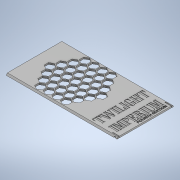
# Autodesk Inventor part: CardboardTray_Lid2
Saved by Autodesk Inventor 2021 (Build 250183000, 183)
## iProperties
Created: 2023-03-19
Part Number: CardboardTray_Lid2
Material: ABS Plastic
Document SubType Name: Modeling
Designer: Bradley
Density: 1.06 g/cm^3
Appearance: Smooth - Medium Gray
Author: Bradley
Autodesk Inventor part; units mm, degrees
(part 1 of 2)
ref_plane "YZ Plane" through (0, 0, 0) normal (1, 0, 0) x (0, 1, 0)
ref_plane "XZ Plane" through (0, 0, 0) normal (0, 1, 0) x (-1, 0, 0)
ref_plane "XY Plane" through (0, 0, 0) normal (0, 0, 1) x (1, 0, 0)
sketch "Sketch1" plane through (0, 0, 0) normal (1, 0, 0) x (0, 1, 0)
  line L0 (-1, 36.1) -> (-1, -36.1)
  line L1 (-1, -36.1) -> (1, -34.6)
  line L2 (1, -34.6) -> (1, 34.6)
  line L3 (1, 34.6) -> (-1, 36.1)
  point P0 (0, 0)
  point P1 (0, 35.35)
  point P2 (1, 0)
  dimension "d0" = 2
  dimension "d1" = 1.5
  dimension "d2" = 69.2
  constraints: 8 end point, 2 midpoint, 1 equal length, 1 horizontal alignment, 1 parallel, 1 vertical, 1 vertical alignment
  measures "d0" distance between parallel lines of L0 L2
  measures "d1" vertical distance of L2.end L0.start
  measures "d2" distance of L1.end L2.end
extrude "Extrusion1" add sketch "Sketch1" along normal mid plane 140.85
sketch "Sketch2" plane through (-70.425, 1, 34.6) normal (0, 1, 0) x (1, 0, 0)
  line L0 (0, 0) -> (140.85, 0) projected
  line L1 (140.85, 69.2) -> (140.85, 0) projected
  line L2 (0, 69.2) -> (140.85, 69.2) projected
  line L3 (0, 0) -> (0, 69.2) projected
  line L4 (0, 69.2) -> (140.85, 69.2) projected
  line L5 (140.85, 70.7) -> (140.85, 69.2) projected
  line L6 (140.85, 70.7) -> (0, 70.7) projected
  line L7 (0, 69.2) -> (0, 70.7) projected
  line L8 (0, -1.5) -> (140.85, -1.5) projected
  line L9 (140.85, 0) -> (140.85, -1.5) projected
  line L10 (0, 0) -> (140.85, 0) projected
  line L11 (0, -1.5) -> (0, 0) projected
  line L12 (140.85, 70.7) -> (0, 70.7) projected
  line L13 (139.1, 70.7) -> (138.8979, 70.35) construction
  line L14 (138.4649, 70.1) -> (137.2351, 70.1) construction
  line L15 (136.8021, 70.35) -> (136.6, 70.7) construction
  arc A0 (138.4649, 70.1) -> (138.8979, 70.35) centre (138.4649, 70.6) ccw construction
  arc A1 (136.8021, 70.35) -> (137.2351, 70.1) centre (137.2351, 70.6) ccw construction
  line L16 (140.35, 70.7) -> (140.85, 70.2)
  line L17 (140.85, 70.7) -> (140.85, 69.2) projected
  line L18 (136.3113, 70.7) -> (136.5856, 70.225)
  arc A2 (136.5856, 70.225) -> (137.2351, 69.85) centre (137.2351, 70.6) ccw
  line L19 (137.2351, 69.85) -> (138.2762, 69.85)
  line L20 (138.9258, 70.225) -> (139.2, 70.7)
  line L21 (0, -1.5) -> (140.85, -1.5) projected
  line L22 (140.35, -1.5) -> (140.85, -1)
  line L23 (140.85, 0) -> (140.85, -1.5) projected
  line L24 (139.2, -1.5) -> (138.9258, -1.025)
  arc A3 (138.9258, -1.025) -> (138.2762, -0.65) centre (138.2762, -1.4) ccw
  line L25 (138.2762, -0.65) -> (137.2351, -0.65)
  arc A4 (137.2351, -0.65) -> (136.5856, -1.025) centre (137.2351, -1.4) ccw
  line L26 (136.5856, -1.025) -> (136.3113, -1.5)
  arc A5 (138.2762, 69.85) -> (138.9258, 70.225) centre (138.2762, 70.6) ccw
  line L27 (140.85, 69.2) -> (140.85, 0) projected
  line L28 (140.85, 68.35) -> (132.85, 68.35)
  arc A6 (132.85, 68.35) -> (132.85, 67.55) centre (132.85, 67.95) ccw
  line L29 (132.85, 67.55) -> (140.85, 67.55)
  line L30 (140.85, 0.85) -> (132.85, 0.85)
  arc A7 (132.85, 1.65) -> (132.85, 0.85) centre (132.85, 1.25) ccw
  line L31 (132.85, 1.65) -> (140.85, 1.65)
  point P0 (70.425, 34.6)
  point P1 (137.7557, -0.65)
  point P2 (137.7557, 69.85)
  point P3 (137.85, 70.1)
  point P4 (140.85, 1.65)
  point P5 (140.85, -1)
  dimension "d5" = 0.5
  dimension "d6" = 45
  dimension "d7" = 0.5
  dimension "d8" = 0.25
  dimension "d10" = 0.6
  dimension "d11" = 60
  dimension "d12" = 2.5
  dimension "d13" = 3
  dimension "d14" = 0.1
  dimension "d15" = 1.5
  dimension "d16" = 0.8
  dimension "d17" = 8
  dimension "d18" = 1.5
  constraints: 30 end point, 16 point on circle, 14 point on line, 14 tangent, 8 centre point, 5 equal length, 5 equal radius, 5 perpendicular, 3 midpoint, 3 vertical alignment, 2 parallel, 1 horizontal, 2 other
  measures "d5" radius of A0
  measures "d6" angle of L6 L16
  measures "d7" horizontal distance of L16.start L16.end
  measures "d8" distance between parallel lines of L19 L14
  measures "d10" distance between parallel lines of L14 L6
  measures "d11" angle of L13 L15
  measures "d12" distance of L13.start L15.end
  measures "d13" distance from line of L17 point (137.85, 70.1)
  measures "d14" distance of L13.start L20.end
  measures "d15" distance between parallel lines of L28 L19
  measures "d16" distance between parallel lines of L29 L28
  measures "d17" distance of L28.start L28.end
  measures "d18" distance between parallel lines of L25 L30
extrude "Extrusion2" cut sketch "Sketch2" against normal through all contours L30 A7 L31 L1 | L9 L8 L22 | L26 A4 L25 A3 L24 L8 | L1 L29 A6 L28 | L16 L6 L5 | L6 L20 A5 L19 A2 L18
sketch "Sketch4" plane through (-70.425, 1, -34.6) normal (0, 1, 0) x (1, 0, 0)
  line L0 (140.85, -68.35) -> (132.85, -68.35) projected
  arc A0 (132.85, -67.55) -> (132.85, -68.35) centre (132.85, -67.95) ccw projected
  line L1 (132.85, -67.55) -> (140.85, -67.55) projected
  line L2 (140.85, -1.65) -> (140.85, -67.55) projected
  line L3 (140.85, -1.65) -> (132.85, -1.65) projected
  arc A1 (132.85, -0.85) -> (132.85, -1.65) centre (132.85, -1.25) ccw projected
  line L4 (132.85, -0.85) -> (140.85, -0.85) projected
  line L5 (140.85, 0) -> (140.85, -0.85) projected
  line L6 (0, 0) -> (140.85, 0) projected
  line L7 (0, -69.2) -> (0, 0) projected
  line L8 (0, -69.2) -> (140.85, -69.2) projected
  line L9 (140.85, -68.35) -> (140.85, -69.2) projected
  line L10 (140.85, -67.55) -> (140.85, -1.65) construction
  line L11 (115.85, 0) -> (115.85, -69.2) construction
  line L12 (0, 1.5) -> (0, -70.7) construction
  line L13 (0, 0) -> (140.85, 0) projected
  line L14 (138.85, -1.65) -> (138.85, -67.55) construction
  line L15 (108.9603, -58.6209) -> (105.0262, -58.6209)
  spline S0 degree 2 poles (105.0262, -58.6209) (104.9674, -58.6209) (104.9185, -58.6894) (104.9185, -58.7481) knots 0 0 0 1 2 2 2
  line L16 (104.9185, -58.7481) -> (104.9185, -66.499)
  spline S1 degree 2 poles (104.9185, -66.499) (104.9185, -66.5577) (104.9674, -66.6262) (105.0262, -66.6262) knots 0 0 0 1 2 2 2
  line L17 (105.0262, -66.6262) -> (108.9603, -66.6262)
  spline S2 degree 2 poles (108.9603, -66.6262) (109.0386, -66.6262) (109.1071, -66.5577) (109.0973, -66.5186) knots 0 0 0 1 2 2 2
  spline S3 degree 2 poles (109.0973, -66.5186) (109.1071, -66.4697) (109.0484, -66.4109) (108.9603, -66.4109) knots 0 0 0 1 2 2 2
  line L18 (108.9603, -66.4109) -> (108.7157, -66.4109)
  spline S4 degree 2 poles (108.7157, -66.4109) (107.7664, -66.4012) (106.1516, -65.8335) (105.1534, -64.8255) (105.1338, -64.1796) knots 0 0 0 1 2 3 3 3
  line L19 (105.1338, -64.1796) -> (105.1338, -63.8958)
  spline S5 degree 2 poles (105.1338, -63.8958) (105.1338, -63.8273) (105.1827, -63.7784) (105.2121, -63.7784) knots 0 0 0 1 2 2 2
  line L20 (105.2121, -63.7784) -> (115.0671, -63.7784)
  spline S6 degree 2 poles (115.0671, -63.7784) (115.439, -63.7686) (115.6738, -63.8371) (115.6641, -63.9448) knots 0 0 0 1 2 2 2
  line L21 (115.6641, -63.9448) -> (115.6641, -64.4243)
  spline S7 degree 2 poles (115.6641, -64.4243) (115.6641, -64.5026) (115.7228, -64.5711) (115.7619, -64.5613) knots 0 0 0 1 2 2 2
  spline S8 degree 2 poles (115.7619, -64.5613) (115.7913, -64.5711) (115.85, -64.5026) (115.85, -64.4243) knots 0 0 0 1 2 2 2
  line L22 (115.85, -64.4243) -> (115.85, -60.8229)
  spline S9 degree 2 poles (115.85, -60.8229) (115.85, -60.7446) (115.7913, -60.6761) (115.7619, -60.6859) knots 0 0 0 1 2 2 2
  spline S10 degree 2 poles (115.7619, -60.6859) (115.7228, -60.6761) (115.6641, -60.7348) (115.6641, -60.8229) knots 0 0 0 1 2 2 2
  line L23 (115.6641, -60.8229) -> (115.6641, -61.3024)
  spline S11 degree 2 poles (115.6641, -61.3024) (115.6738, -61.4003) (115.439, -61.4688) (115.0671, -61.4688) knots 0 0 0 1 2 2 2
  line L24 (115.0671, -61.4688) -> (105.2121, -61.4688)
  spline S12 degree 2 poles (105.2121, -61.4688) (105.1827, -61.4688) (105.1338, -61.4101) (105.1338, -61.3318) knots 0 0 0 1 2 2 2
  line L25 (105.1338, -61.3318) -> (105.1338, -61.0675)
  spline S13 degree 2 poles (105.1338, -61.0675) (105.1534, -60.4216) (106.1516, -59.4136) (107.7664, -58.846) (108.7157, -58.8362) knots 0 0 0 1 2 3 3 3
  line L26 (108.7157, -58.8362) -> (108.9603, -58.8362)
  spline S14 degree 2 poles (108.9603, -58.8362) (109.0484, -58.8362) (109.1071, -58.7775) (109.0973, -58.7286) knots 0 0 0 1 2 2 2
  spline S15 degree 2 poles (109.0973, -58.7286) (109.1071, -58.6796) (109.0386, -58.6209) (108.9603, -58.6209) knots 0 0 0 1 2 2 2
  spline S16 degree 2 poles (105.0164, -44.7828) (104.9772, -44.7828) (104.9185, -44.8318) (104.9185, -44.9198) knots 0 0 0 1 2 2 2
  line L27 (104.9185, -44.9198) -> (104.9185, -47.3371)
  spline S17 degree 2 poles (104.9185, -47.3371) (104.9185, -47.4154) (104.9772, -47.4643) (105.0164, -47.4643) knots 0 0 0 1 2 2 2
  spline S18 degree 2 poles (105.0164, -47.4643) (105.0457, -47.4643) (105.1044, -47.4154) (105.1044, -47.3371) knots 0 0 0 1 2 2 2
  line L28 (105.1044, -47.3371) -> (105.1044, -47.1512)
  spline S19 degree 2 poles (105.1044, -47.1512) (105.1142, -46.6129) (106.5333, -46.2606) (107.874, -46.5346) knots 0 0 0 1 2 2 2
  line L29 (107.874, -46.5346) -> (113.9319, -47.7873)
  line L30 (113.9319, -47.7873) -> (113.9319, -47.8362)
  line L31 (113.9319, -47.8362) -> (105.7406, -49.6271)
  spline S20 degree 2 poles (105.7406, -49.6271) (105.3295, -49.725) (105.0947, -49.6467) (105.1044, -49.4999) knots 0 0 0 1 2 2 2
  line L32 (105.1044, -49.4999) -> (105.1044, -49.128)
  spline S21 degree 2 poles (105.1044, -49.128) (105.1044, -49.0399) (105.0457, -48.991) (105.0164, -48.991) knots 0 0 0 1 2 2 2
  spline S22 degree 2 poles (105.0164, -48.991) (104.9772, -48.991) (104.9185, -49.0399) (104.9185, -49.128) knots 0 0 0 1 2 2 2
  line L33 (104.9185, -49.128) -> (104.9185, -52.8273)
  spline S23 degree 2 poles (104.9185, -52.8273) (104.9185, -52.9154) (104.9772, -52.9741) (105.0164, -52.9741) knots 0 0 0 1 2 2 2
  spline S24 degree 2 poles (105.0164, -52.9741) (105.0457, -52.9741) (105.1044, -52.9252) (105.1044, -52.8273) knots 0 0 0 1 2 2 2
  line L34 (105.1044, -52.8273) -> (105.1044, -52.6609)
  spline S25 degree 2 poles (105.1044, -52.6609) (105.1142, -52.1129) (106.5333, -51.7802) (107.874, -52.0444) knots 0 0 0 1 2 2 2
  line L35 (107.874, -52.0444) -> (113.9319, -53.2383)
  line L36 (113.9319, -53.2383) -> (113.9319, -53.2775)
  line L37 (113.9319, -53.2775) -> (105.7406, -55.1369)
  spline S26 degree 2 poles (105.7406, -55.1369) (105.3393, -55.225) (105.0947, -55.1565) (105.1044, -55.0097) knots 0 0 0 1 2 2 2
  line L38 (105.1044, -55.0097) -> (105.1044, -54.628)
  spline S27 degree 2 poles (105.1044, -54.628) (105.1044, -54.5399) (105.0457, -54.4812) (105.0164, -54.491) knots 0 0 0 1 2 2 2
  spline S28 degree 2 poles (105.0164, -54.491) (104.9772, -54.4812) (104.9185, -54.5497) (104.9185, -54.628) knots 0 0 0 1 2 2 2
  line L39 (104.9185, -54.628) -> (104.9185, -58.1903)
  spline S29 degree 2 poles (104.9185, -58.1903) (104.9185, -58.2686) (104.9772, -58.3273) (105.0164, -58.3273) knots 0 0 0 1 2 2 2
  spline S30 degree 2 poles (105.0164, -58.3273) (105.0457, -58.3273) (105.1044, -58.2784) (105.1044, -58.1903) knots 0 0 0 1 2 2 2
  line L40 (105.1044, -58.1903) -> (105.1044, -57.9848)
  spline S31 degree 2 poles (105.1044, -57.9848) (105.0947, -57.8576) (105.3393, -57.701) (105.7406, -57.6031) knots 0 0 0 1 2 2 2
  line L41 (105.7406, -57.6031) -> (115.7913, -55.1076)
  spline S32 degree 2 poles (115.7913, -55.1076) (115.8304, -55.1076) (115.8794, -55.0586) (115.8794, -54.9999) knots 0 0 0 1 2 2 2
  line L42 (115.8794, -54.9999) -> (115.8794, -53.5613)
  spline S33 degree 2 poles (115.8794, -53.5613) (115.8794, -53.4928) (115.8304, -53.4439) (115.7913, -53.4341) knots 0 0 0 1 2 2 2
  line L43 (115.7913, -53.4341) -> (107.5413, -51.7019)
  line L44 (107.5413, -51.7019) -> (107.5413, -51.6725)
  line L45 (107.5413, -51.6725) -> (115.7913, -49.6565)
  spline S34 degree 2 poles (115.7913, -49.6565) (115.8304, -49.6565) (115.8794, -49.6076) (115.8794, -49.5488) knots 0 0 0 1 2 2 2
  line L46 (115.8794, -49.5488) -> (115.8794, -48.1102)
  spline S35 degree 2 poles (115.8794, -48.1102) (115.8794, -48.0417) (115.8304, -47.9928) (115.7913, -47.983) knots 0 0 0 1 2 2 2
  line L47 (115.7913, -47.983) -> (108.0306, -46.3193)
  spline S36 degree 2 poles (108.0306, -46.3193) (106.7388, -46.0257) (105.4763, -45.5364) (105.0849, -45.1254) (105.1044, -44.9492) knots 0 0 0 1 2 3 3 3
  line L48 (105.1044, -44.9492) -> (105.1044, -44.9198)
  spline S37 degree 2 poles (105.1044, -44.9198) (105.1044, -44.8318) (105.0457, -44.7828) (105.0164, -44.7828) knots 0 0 0 1 2 2 2
  spline S38 degree 2 poles (115.7619, -40.6921) (115.7228, -40.6823) (115.6641, -40.741) (115.6641, -40.8291) knots 0 0 0 1 2 2 2
  line L49 (115.6641, -40.8291) -> (115.6641, -41.2597)
  spline S39 degree 2 poles (115.6641, -41.2597) (115.6738, -41.3673) (115.439, -41.4163) (115.0671, -41.4163) knots 0 0 0 1 2 2 2
  line L50 (115.0671, -41.4163) -> (105.7112, -41.4163)
  spline S40 degree 2 poles (105.7112, -41.4163) (105.3393, -41.4163) (105.0947, -41.3673) (105.1044, -41.2597) knots 0 0 0 1 2 2 2
  line L51 (105.1044, -41.2597) -> (105.1044, -40.8291)
  spline S41 degree 2 poles (105.1044, -40.8291) (105.1044, -40.741) (105.0457, -40.6823) (105.0164, -40.6921) knots 0 0 0 1 2 2 2
  spline S42 degree 2 poles (105.0164, -40.6921) (104.9772, -40.6921) (104.9185, -40.7508) (104.9185, -40.8291) knots 0 0 0 1 2 2 2
  line L52 (104.9185, -40.8291) -> (104.9185, -44.3229)
  spline S43 degree 2 poles (104.9185, -44.3229) (104.9185, -44.4012) (104.9772, -44.4599) (105.0164, -44.4599) knots 0 0 0 1 2 2 2
  spline S44 degree 2 poles (105.0164, -44.4599) (105.0457, -44.4697) (105.1044, -44.4109) (105.1044, -44.3229) knots 0 0 0 1 2 2 2
  line L53 (105.1044, -44.3229) -> (105.1044, -43.8923)
  spline S45 degree 2 poles (105.1044, -43.8923) (105.0947, -43.7846) (105.3393, -43.7357) (105.7112, -43.7357) knots 0 0 0 1 2 2 2
  line L54 (105.7112, -43.7357) -> (115.0671, -43.7357)
  spline S46 degree 2 poles (115.0671, -43.7357) (115.439, -43.7357) (115.6738, -43.7846) (115.6641, -43.8923) knots 0 0 0 1 2 2 2
  line L55 (115.6641, -43.8923) -> (115.6641, -44.3229)
  spline S47 degree 2 poles (115.6641, -44.3229) (115.6641, -44.4109) (115.7228, -44.4697) (115.7619, -44.4599) knots 0 0 0 1 2 2 2
  spline S48 degree 2 poles (115.7619, -44.4599) (115.7913, -44.4599) (115.85, -44.4012) (115.85, -44.3229) knots 0 0 0 1 2 2 2
  line L56 (115.85, -44.3229) -> (115.85, -40.8291)
  spline S49 degree 2 poles (115.85, -40.8291) (115.85, -40.7508) (115.7913, -40.6921) (115.7619, -40.6921) knots 0 0 0 1 2 2 2
  line L57 (115.7228, -33.2935) -> (111.5929, -33.2935)
  spline S50 degree 2 poles (111.5929, -33.2935) (111.5048, -33.2935) (111.4559, -33.362) (111.4559, -33.4109) knots 0 0 0 1 2 2 2
  spline S51 degree 2 poles (111.4559, -33.4109) (111.4559, -33.4501) (111.5048, -33.5088) (111.5929, -33.5088) knots 0 0 0 1 2 2 2
  line L58 (111.5929, -33.5088) -> (111.8278, -33.5088)
  spline S52 degree 2 poles (111.8278, -33.5088) (112.3367, -33.5088) (113.6187, -33.8122) (114.8322, -34.4777) (115.6249, -35.564) (115.6347, -36.3567) knots 0 0 0 1 2 3 4 4 4
  line L59 (115.6347, -36.3567) -> (115.6347, -36.9439)
  spline S53 degree 2 poles (115.6347, -36.9439) (115.6347, -37.0124) (115.5956, -37.0515) (115.5564, -37.0515) knots 0 0 0 1 2 2 2
  line L60 (115.5564, -37.0515) -> (105.7112, -37.0515)
  spline S54 degree 2 poles (105.7112, -37.0515) (105.3393, -37.0515) (105.0947, -37.0026) (105.1044, -36.8949) knots 0 0 0 1 2 2 2
  line L61 (105.1044, -36.8949) -> (105.1044, -36.1903)
  spline S55 degree 2 poles (105.1044, -36.1903) (105.1044, -36.0924) (105.0457, -36.0435) (105.0164, -36.0435) knots 0 0 0 1 2 2 2
  spline S56 degree 2 poles (105.0164, -36.0435) (104.9772, -36.0435) (104.9185, -36.0924) (104.9185, -36.1903) knots 0 0 0 1 2 2 2
  line L62 (104.9185, -36.1903) -> (104.9185, -39.9581)
  spline S57 degree 2 poles (104.9185, -39.9581) (104.9185, -40.0364) (104.9772, -40.0951) (105.0164, -40.0951) knots 0 0 0 1 2 2 2
  spline S58 degree 2 poles (105.0164, -40.0951) (105.0457, -40.1049) (105.1044, -40.0462) (105.1044, -39.9581) knots 0 0 0 1 2 2 2
  line L63 (105.1044, -39.9581) -> (105.1044, -39.5275)
  spline S59 degree 2 poles (105.1044, -39.5275) (105.0947, -39.4198) (105.3393, -39.3709) (105.7112, -39.3709) knots 0 0 0 1 2 2 2
  line L64 (105.7112, -39.3709) -> (115.0671, -39.3709)
  spline S60 degree 2 poles (115.0671, -39.3709) (115.439, -39.3709) (115.6738, -39.4198) (115.6641, -39.5275) knots 0 0 0 1 2 2 2
  line L65 (115.6641, -39.5275) -> (115.6641, -39.9581)
  spline S61 degree 2 poles (115.6641, -39.9581) (115.6641, -40.0462) (115.7228, -40.1049) (115.7619, -40.0951) knots 0 0 0 1 2 2 2
  spline S62 degree 2 poles (115.7619, -40.0951) (115.7913, -40.0951) (115.85, -40.0364) (115.85, -39.9581) knots 0 0 0 1 2 2 2
  line L66 (115.85, -39.9581) -> (115.85, -33.4109)
  spline S63 degree 2 poles (115.85, -33.4109) (115.85, -33.3522) (115.7913, -33.2935) (115.7228, -33.2935) knots 0 0 0 1 2 2 2
  spline S64 degree 2 poles (115.7619, -28.7917) (115.7228, -28.7819) (115.6641, -28.8407) (115.6641, -28.9287) knots 0 0 0 1 2 2 2
  line L67 (115.6641, -28.9287) -> (115.6641, -29.3593)
  spline S65 degree 2 poles (115.6641, -29.3593) (115.6738, -29.467) (115.439, -29.5159) (115.0671, -29.5159) knots 0 0 0 1 2 2 2
  line L68 (115.0671, -29.5159) -> (105.7112, -29.5159)
  spline S66 degree 2 poles (105.7112, -29.5159) (105.3393, -29.5159) (105.0947, -29.467) (105.1044, -29.3593) knots 0 0 0 1 2 2 2
  line L69 (105.1044, -29.3593) -> (105.1044, -28.9287)
  spline S67 degree 2 poles (105.1044, -28.9287) (105.1044, -28.8407) (105.0457, -28.7819) (105.0164, -28.7917) knots 0 0 0 1 2 2 2
  spline S68 degree 2 poles (105.0164, -28.7917) (104.9772, -28.7917) (104.9185, -28.8504) (104.9185, -28.9287) knots 0 0 0 1 2 2 2
  line L70 (104.9185, -28.9287) -> (104.9185, -32.4225)
  spline S69 degree 2 poles (104.9185, -32.4225) (104.9185, -32.5008) (104.9772, -32.5595) (105.0164, -32.5595) knots 0 0 0 1 2 2 2
  spline S70 degree 2 poles (105.0164, -32.5595) (105.0457, -32.5693) (105.1044, -32.5106) (105.1044, -32.4225) knots 0 0 0 1 2 2 2
  line L71 (105.1044, -32.4225) -> (105.1044, -31.9919)
  spline S71 degree 2 poles (105.1044, -31.9919) (105.0947, -31.8843) (105.3393, -31.8353) (105.7112, -31.8353) knots 0 0 0 1 2 2 2
  line L72 (105.7112, -31.8353) -> (115.0671, -31.8353)
  spline S72 degree 2 poles (115.0671, -31.8353) (115.439, -31.8353) (115.6738, -31.8843) (115.6641, -31.9919) knots 0 0 0 1 2 2 2
  line L73 (115.6641, -31.9919) -> (115.6641, -32.4225)
  spline S73 degree 2 poles (115.6641, -32.4225) (115.6641, -32.5106) (115.7228, -32.5693) (115.7619, -32.5595) knots 0 0 0 1 2 2 2
  spline S74 degree 2 poles (115.7619, -32.5595) (115.7913, -32.5595) (115.85, -32.5008) (115.85, -32.4225) knots 0 0 0 1 2 2 2
  line L74 (115.85, -32.4225) -> (115.85, -28.9287)
  spline S75 degree 2 poles (115.85, -28.9287) (115.85, -28.8504) (115.7913, -28.7917) (115.7619, -28.7917) knots 0 0 0 1 2 2 2
  spline S76 degree 2 poles (111.2406, -20.1013) (111.2014, -20.0915) (111.1427, -20.1601) (111.1427, -20.2383) knots 0 0 0 1 2 2 2
  line L75 (111.1427, -20.2383) -> (111.1427, -24.0746)
  spline S77 degree 2 poles (111.1427, -24.0746) (111.1427, -24.1725) (111.2014, -24.2214) (111.2406, -24.2214) knots 0 0 0 1 2 2 2
  spline S78 degree 2 poles (111.2406, -24.2214) (111.2699, -24.2214) (111.3286, -24.1725) (111.3286, -24.0746) knots 0 0 0 1 2 2 2
  line L76 (111.3286, -24.0746) -> (111.3286, -23.2428)
  spline S79 degree 2 poles (111.3286, -23.2428) (111.3189, -23.1351) (111.5635, -23.0764) (111.9354, -23.0862) knots 0 0 0 1 2 2 2
  line L77 (111.9354, -23.0862) -> (114.1961, -23.0862)
  spline S80 degree 2 poles (114.1961, -23.0862) (114.9888, -23.0666) (115.8598, -23.4972) (115.8696, -24.1431) knots 0 0 0 1 2 2 2
  spline S81 degree 2 poles (115.8696, -24.1431) (115.8598, -24.7108) (115.0769, -25.2099) (113.648, -25.3371) (112.6792, -25.3665) knots 0 0 0 1 2 3 3 3
  spline S82 degree 2 poles (112.6792, -25.3665) (111.544, -25.4154) (109.2833, -25.4154) (108.1578, -25.3665) knots 0 0 0 1 2 2 2
  spline S83 degree 2 poles (108.1578, -25.3665) (107.2966, -25.3469) (105.8286, -25.2001) (104.9185, -24.6716) (104.9087, -24.0942) knots 0 0 0 1 2 3 3 3
  spline S84 degree 2 poles (104.9087, -24.0942) (104.9185, -23.5462) (105.8286, -22.4403) (107.5315, -21.6867) (108.7352, -21.677) knots 0 0 0 1 2 3 3 3
  line L78 (108.7352, -21.677) -> (108.9016, -21.677)
  spline S85 degree 2 poles (108.9016, -21.677) (108.9897, -21.677) (109.0386, -21.6182) (109.0386, -21.5791) knots 0 0 0 1 2 2 2
  spline S86 degree 2 poles (109.0386, -21.5791) (109.0386, -21.5302) (108.9897, -21.4617) (108.9016, -21.4617) knots 0 0 0 1 2 2 2
  line L79 (108.9016, -21.4617) -> (105.0359, -21.4617)
  spline S87 degree 2 poles (105.0359, -21.4617) (104.9479, -21.4617) (104.8794, -21.5302) (104.8794, -21.5791) knots 0 0 0 1 2 2 2
  spline S88 degree 2 poles (104.8794, -21.5791) (104.8794, -21.6182) (104.9479, -21.677) (105.0359, -21.677) knots 0 0 0 1 2 2 2
  line L80 (105.0359, -21.677) -> (105.1436, -21.677)
  spline S89 degree 2 poles (105.1436, -21.677) (105.398, -21.6867) (105.2806, -22.1076) (105.1534, -22.3522) knots 0 0 0 1 2 2 2
  spline S90 degree 2 poles (105.1534, -22.3522) (105.0164, -22.6556) (104.7326, -23.5951) (104.7228, -24.1236) knots 0 0 0 1 2 2 2
  spline S91 degree 2 poles (104.7228, -24.1236) (104.7423, -25.4154) (106.2593, -27.177) (108.8625, -28.0871) (110.4968, -28.0871) knots 0 0 0 1 2 3 3 3
  spline S92 degree 2 poles (110.4968, -28.0871) (111.4657, -28.0871) (113.4132, -27.6663) (115.0377, -26.7366) (116.0262, -25.249) (116.0359, -24.1823) knots 0 0 0 1 2 3 4 4 4
  spline S93 degree 2 poles (116.0359, -24.1823) (116.0262, -23.6147) (115.6836, -22.8122) (115.3411, -22.0684) (115.3215, -21.5693) knots 0 0 0 1 2 3 3 3
  spline S94 degree 2 poles (115.3215, -21.5693) (115.3313, -21.2757) (115.5075, -20.9919) (115.6543, -20.9919) knots 0 0 0 1 2 2 2
  line L81 (115.6543, -20.9919) -> (115.7326, -20.9919)
  spline S95 degree 2 poles (115.7326, -20.9919) (115.8206, -20.9919) (115.8794, -20.9234) (115.8794, -20.8745) knots 0 0 0 1 2 2 2
  spline S96 degree 2 poles (115.8794, -20.8745) (115.8794, -20.8353) (115.8206, -20.7766) (115.7326, -20.7766) knots 0 0 0 1 2 2 2
  line L82 (115.7326, -20.7766) -> (111.9354, -20.7766)
  spline S97 degree 2 poles (111.9354, -20.7766) (111.5635, -20.7766) (111.3189, -20.7081) (111.3286, -20.6102) knots 0 0 0 1 2 2 2
  line L83 (111.3286, -20.6102) -> (111.3286, -20.2383)
  spline S98 degree 2 poles (111.3286, -20.2383) (111.3286, -20.1503) (111.2699, -20.0915) (111.2406, -20.1013) knots 0 0 0 1 2 2 2
  spline S99 degree 2 poles (115.7619, -11.1565) (115.7228, -11.1565) (115.6641, -11.2054) (115.6641, -11.2935) knots 0 0 0 1 2 2 2
  line L84 (115.6641, -11.2935) -> (115.6641, -11.7143)
  spline S100 degree 2 poles (115.6641, -11.7143) (115.6738, -11.822) (115.439, -11.8905) (115.0671, -11.8807) knots 0 0 0 1 2 2 2
  line L85 (115.0671, -11.8807) -> (105.7112, -11.8807)
  spline S101 degree 2 poles (105.7112, -11.8807) (105.3393, -11.8807) (105.0947, -11.8122) (105.1044, -11.7143) knots 0 0 0 1 2 2 2
  line L86 (105.1044, -11.7143) -> (105.1044, -11.2739)
  spline S102 degree 2 poles (105.1044, -11.2739) (105.1044, -11.1956) (105.0457, -11.1369) (105.0164, -11.1369) knots 0 0 0 1 2 2 2
  spline S103 degree 2 poles (105.0164, -11.1369) (104.9772, -11.1369) (104.9185, -11.1956) (104.9185, -11.2739) knots 0 0 0 1 2 2 2
  line L87 (104.9185, -11.2739) -> (104.9185, -14.7775)
  spline S104 degree 2 poles (104.9185, -14.7775) (104.9185, -14.8656) (104.9772, -14.9243) (105.0164, -14.9145) knots 0 0 0 1 2 2 2
  spline S105 degree 2 poles (105.0164, -14.9145) (105.0457, -14.9243) (105.1044, -14.8656) (105.1044, -14.7775) knots 0 0 0 1 2 2 2
  line L88 (105.1044, -14.7775) -> (105.1044, -14.3567)
  spline S106 degree 2 poles (105.1044, -14.3567) (105.0947, -14.249) (105.3393, -14.1805) (105.7112, -14.1903) knots 0 0 0 1 2 2 2
  line L89 (105.7112, -14.1903) -> (109.9977, -14.1903)
  spline S107 degree 2 poles (109.9977, -14.1903) (110.0368, -14.1903) (110.1053, -14.2392) (110.1053, -14.3175) knots 0 0 0 1 2 2 2
  line L90 (110.1053, -14.3175) -> (110.1053, -16.4999)
  spline S108 degree 2 poles (110.1053, -16.4999) (110.1053, -16.5684) (110.0368, -16.6076) (109.9977, -16.6076) knots 0 0 0 1 2 2 2
  line L91 (109.9977, -16.6076) -> (105.7112, -16.6076)
  spline S109 degree 2 poles (105.7112, -16.6076) (105.3393, -16.6076) (105.0947, -16.5586) (105.1044, -16.451) knots 0 0 0 1 2 2 2
  line L92 (105.1044, -16.451) -> (105.1044, -16.0204)
  spline S110 degree 2 poles (105.1044, -16.0204) (105.1044, -15.9323) (105.0457, -15.8736) (105.0164, -15.8834) knots 0 0 0 1 2 2 2
  spline S111 degree 2 poles (105.0164, -15.8834) (104.9772, -15.8736) (104.9185, -15.9421) (104.9185, -16.0204) knots 0 0 0 1 2 2 2
  line L93 (104.9185, -16.0204) -> (104.9185, -19.5141)
  spline S112 degree 2 poles (104.9185, -19.5141) (104.9185, -19.5924) (104.9772, -19.6512) (105.0164, -19.6512) knots 0 0 0 1 2 2 2
  spline S113 degree 2 poles (105.0164, -19.6512) (105.0457, -19.6609) (105.1044, -19.6022) (105.1044, -19.5141) knots 0 0 0 1 2 2 2
  line L94 (105.1044, -19.5141) -> (105.1044, -19.0835)
  spline S114 degree 2 poles (105.1044, -19.0835) (105.0947, -18.9759) (105.3393, -18.927) (105.7112, -18.927) knots 0 0 0 1 2 2 2
  line L95 (105.7112, -18.927) -> (115.0671, -18.927)
  spline S115 degree 2 poles (115.0671, -18.927) (115.439, -18.927) (115.6738, -18.9759) (115.6641, -19.0835) knots 0 0 0 1 2 2 2
  line L96 (115.6641, -19.0835) -> (115.6641, -19.5141)
  spline S116 degree 2 poles (115.6641, -19.5141) (115.6641, -19.6022) (115.7228, -19.6609) (115.7619, -19.6512) knots 0 0 0 1 2 2 2
  spline S117 degree 2 poles (115.7619, -19.6512) (115.7913, -19.6512) (115.85, -19.5924) (115.85, -19.5141) knots 0 0 0 1 2 2 2
  line L97 (115.85, -19.5141) -> (115.85, -16.0204)
  spline S118 degree 2 poles (115.85, -16.0204) (115.85, -15.9421) (115.7913, -15.8736) (115.7619, -15.8834) knots 0 0 0 1 2 2 2
  spline S119 degree 2 poles (115.7619, -15.8834) (115.7228, -15.8736) (115.6641, -15.9323) (115.6641, -16.0204) knots 0 0 0 1 2 2 2
  line L98 (115.6641, -16.0204) -> (115.6641, -16.451)
  spline S120 degree 2 poles (115.6641, -16.451) (115.6738, -16.5586) (115.439, -16.6076) (115.0671, -16.6076) knots 0 0 0 1 2 2 2
  line L99 (115.0671, -16.6076) -> (110.3989, -16.6076)
  spline S121 degree 2 poles (110.3989, -16.6076) (110.3598, -16.6076) (110.2913, -16.5684) (110.2913, -16.4999) knots 0 0 0 1 2 2 2
  line L100 (110.2913, -16.4999) -> (110.2913, -14.3175)
  spline S122 degree 2 poles (110.2913, -14.3175) (110.2913, -14.2392) (110.3598, -14.1903) (110.3989, -14.1903) knots 0 0 0 1 2 2 2
  line L101 (110.3989, -14.1903) -> (115.0671, -14.1903)
  spline S123 degree 2 poles (115.0671, -14.1903) (115.439, -14.1805) (115.6738, -14.249) (115.6641, -14.3567) knots 0 0 0 1 2 2 2
  line L102 (115.6641, -14.3567) -> (115.6641, -14.7775)
  spline S124 degree 2 poles (115.6641, -14.7775) (115.6641, -14.8656) (115.7228, -14.9243) (115.7619, -14.9145) knots 0 0 0 1 2 2 2
  spline S125 degree 2 poles (115.7619, -14.9145) (115.7913, -14.9243) (115.85, -14.8656) (115.85, -14.7775) knots 0 0 0 1 2 2 2
  line L103 (115.85, -14.7775) -> (115.85, -11.2935)
  spline S126 degree 2 poles (115.85, -11.2935) (115.85, -11.2054) (115.7913, -11.1565) (115.7619, -11.1565) knots 0 0 0 1 2 2 2
  line L104 (108.9603, -2.5933) -> (105.0262, -2.5933)
  spline S127 degree 2 poles (105.0262, -2.5933) (104.9674, -2.5933) (104.9185, -2.6618) (104.9185, -2.7206) knots 0 0 0 1 2 2 2
  line L105 (104.9185, -2.7206) -> (104.9185, -10.4714)
  spline S128 degree 2 poles (104.9185, -10.4714) (104.9185, -10.5302) (104.9674, -10.5987) (105.0262, -10.5987) knots 0 0 0 1 2 2 2
  line L106 (105.0262, -10.5987) -> (108.9603, -10.5987)
  spline S129 degree 2 poles (108.9603, -10.5987) (109.0386, -10.5987) (109.1071, -10.5302) (109.0973, -10.491) knots 0 0 0 1 2 2 2
  spline S130 degree 2 poles (109.0973, -10.491) (109.1071, -10.4421) (109.0484, -10.3834) (108.9603, -10.3834) knots 0 0 0 1 2 2 2
  line L107 (108.9603, -10.3834) -> (108.7157, -10.3834)
  spline S131 degree 2 poles (108.7157, -10.3834) (107.7664, -10.3736) (106.1516, -9.806) (105.1534, -8.798) (105.1338, -8.152) knots 0 0 0 1 2 3 3 3
  line L108 (105.1338, -8.152) -> (105.1338, -7.8682)
  spline S132 degree 2 poles (105.1338, -7.8682) (105.1338, -7.7997) (105.1827, -7.7508) (105.2121, -7.7508) knots 0 0 0 1 2 2 2
  line L109 (105.2121, -7.7508) -> (115.0671, -7.7508)
  spline S133 degree 2 poles (115.0671, -7.7508) (115.439, -7.741) (115.6738, -7.8095) (115.6641, -7.9172) knots 0 0 0 1 2 2 2
  line L110 (115.6641, -7.9172) -> (115.6641, -8.3967)
  spline S134 degree 2 poles (115.6641, -8.3967) (115.6641, -8.475) (115.7228, -8.5435) (115.7619, -8.5337) knots 0 0 0 1 2 2 2
  spline S135 degree 2 poles (115.7619, -8.5337) (115.7913, -8.5435) (115.85, -8.475) (115.85, -8.3967) knots 0 0 0 1 2 2 2
  line L111 (115.85, -8.3967) -> (115.85, -4.7953)
  spline S136 degree 2 poles (115.85, -4.7953) (115.85, -4.717) (115.7913, -4.6485) (115.7619, -4.6583) knots 0 0 0 1 2 2 2
  spline S137 degree 2 poles (115.7619, -4.6583) (115.7228, -4.6485) (115.6641, -4.7072) (115.6641, -4.7953) knots 0 0 0 1 2 2 2
  line L112 (115.6641, -4.7953) -> (115.6641, -5.2748)
  spline S138 degree 2 poles (115.6641, -5.2748) (115.6738, -5.3727) (115.439, -5.4412) (115.0671, -5.4412) knots 0 0 0 1 2 2 2
  line L113 (115.0671, -5.4412) -> (105.2121, -5.4412)
  spline S139 degree 2 poles (105.2121, -5.4412) (105.1827, -5.4412) (105.1338, -5.3825) (105.1338, -5.3042) knots 0 0 0 1 2 2 2
  line L114 (105.1338, -5.3042) -> (105.1338, -5.0399)
  spline S140 degree 2 poles (105.1338, -5.0399) (105.1534, -4.394) (106.1516, -3.386) (107.7664, -2.8184) (108.7157, -2.8086) knots 0 0 0 1 2 3 3 3
  line L115 (108.7157, -2.8086) -> (108.9603, -2.8086)
  spline S141 degree 2 poles (108.9603, -2.8086) (109.0484, -2.8086) (109.1071, -2.7499) (109.0973, -2.701) knots 0 0 0 1 2 2 2
  spline S142 degree 2 poles (109.0973, -2.701) (109.1071, -2.652) (109.0386, -2.5933) (108.9603, -2.5933) knots 0 0 0 1 2 2 2
  spline S143 degree 2 poles (134.4921, -60.9795) (134.4529, -60.9697) (134.3942, -61.0284) (134.3942, -61.1165) knots 0 0 0 1 2 2 2
  line L116 (134.3942, -61.1165) -> (134.3942, -61.5471)
  spline S144 degree 2 poles (134.3942, -61.5471) (134.404, -61.6547) (134.1691, -61.7036) (133.7972, -61.7036) knots 0 0 0 1 2 2 2
  line L117 (133.7972, -61.7036) -> (124.4414, -61.7036)
  spline S145 degree 2 poles (124.4414, -61.7036) (124.0695, -61.7036) (123.8248, -61.6547) (123.8346, -61.5471) knots 0 0 0 1 2 2 2
  line L118 (123.8346, -61.5471) -> (123.8346, -61.1165)
  spline S146 degree 2 poles (123.8346, -61.1165) (123.8346, -61.0284) (123.7759, -60.9697) (123.7465, -60.9795) knots 0 0 0 1 2 2 2
  spline S147 degree 2 poles (123.7465, -60.9795) (123.7074, -60.9795) (123.6487, -61.0382) (123.6487, -61.1165) knots 0 0 0 1 2 2 2
  line L119 (123.6487, -61.1165) -> (123.6487, -64.6102)
  spline S148 degree 2 poles (123.6487, -64.6102) (123.6487, -64.6885) (123.7074, -64.7472) (123.7465, -64.7472) knots 0 0 0 1 2 2 2
  spline S149 degree 2 poles (123.7465, -64.7472) (123.7759, -64.757) (123.8346, -64.6983) (123.8346, -64.6102) knots 0 0 0 1 2 2 2
  line L120 (123.8346, -64.6102) -> (123.8346, -64.1796)
  spline S150 degree 2 poles (123.8346, -64.1796) (123.8248, -64.072) (124.0695, -64.023) (124.4414, -64.023) knots 0 0 0 1 2 2 2
  line L121 (124.4414, -64.023) -> (133.7972, -64.023)
  spline S151 degree 2 poles (133.7972, -64.023) (134.1691, -64.023) (134.404, -64.072) (134.3942, -64.1796) knots 0 0 0 1 2 2 2
  line L122 (134.3942, -64.1796) -> (134.3942, -64.6102)
  spline S152 degree 2 poles (134.3942, -64.6102) (134.3942, -64.6983) (134.4529, -64.757) (134.4921, -64.7472) knots 0 0 0 1 2 2 2
  spline S153 degree 2 poles (134.4921, -64.7472) (134.5214, -64.7472) (134.5802, -64.6885) (134.5802, -64.6102) knots 0 0 0 1 2 2 2
  line L123 (134.5802, -64.6102) -> (134.5802, -61.1165)
  spline S154 degree 2 poles (134.5802, -61.1165) (134.5802, -61.0382) (134.5214, -60.9795) (134.4921, -60.9795) knots 0 0 0 1 2 2 2
  spline S155 degree 2 poles (134.4921, -51.0266) (134.4529, -51.0168) (134.3942, -51.0755) (134.3942, -51.1636) knots 0 0 0 1 2 2 2
  line L124 (134.3942, -51.1636) -> (134.3942, -51.5942)
  spline S156 degree 2 poles (134.3942, -51.5942) (134.404, -51.7019) (134.1691, -51.7508) (133.7972, -51.7508) knots 0 0 0 1 2 2 2
  line L125 (133.7972, -51.7508) -> (124.4414, -51.7508)
  spline S157 degree 2 poles (124.4414, -51.7508) (124.0695, -51.7508) (123.8248, -51.7019) (123.8346, -51.5942) knots 0 0 0 1 2 2 2
  line L126 (123.8346, -51.5942) -> (123.8346, -51.1636)
  spline S158 degree 2 poles (123.8346, -51.1636) (123.8346, -51.0755) (123.7759, -51.0168) (123.7465, -51.0266) knots 0 0 0 1 2 2 2
  spline S159 degree 2 poles (123.7465, -51.0266) (123.7074, -51.0266) (123.6487, -51.0853) (123.6487, -51.1636) knots 0 0 0 1 2 2 2
  line L127 (123.6487, -51.1636) -> (123.6487, -54.0506)
  spline S160 degree 2 poles (123.6487, -54.0506) (123.6487, -54.1387) (123.7172, -54.2072) (123.7759, -54.2072) knots 0 0 0 1 2 2 2
  line L128 (123.7759, -54.2072) -> (131.9182, -55.5675)
  line L129 (131.9182, -55.5675) -> (131.9182, -55.5871)
  line L130 (131.9182, -55.5871) -> (123.7759, -57.1138)
  spline S161 degree 2 poles (123.7759, -57.1138) (123.7172, -57.1334) (123.6487, -57.2214) (123.6487, -57.2899) knots 0 0 0 1 2 2 2
  line L131 (123.6487, -57.2899) -> (123.6487, -60.2944)
  spline S162 degree 2 poles (123.6487, -60.2944) (123.6487, -60.3727) (123.7074, -60.4216) (123.7465, -60.4118) knots 0 0 0 1 2 2 2
  spline S163 degree 2 poles (123.7465, -60.4118) (123.7759, -60.4216) (123.8346, -60.3727) (123.8346, -60.2944) knots 0 0 0 1 2 2 2
  line L132 (123.8346, -60.2944) -> (123.8346, -59.7953)
  spline S164 degree 2 poles (123.8346, -59.7953) (123.8248, -59.6974) (124.0695, -59.6387) (124.4414, -59.6387) knots 0 0 0 1 2 2 2
  line L133 (124.4414, -59.6387) -> (130.9004, -59.6387)
  spline S165 degree 2 poles (130.9004, -59.6387) (132.2608, -59.6387) (133.7972, -59.7757) (134.404, -60.0889) (134.3942, -60.3531) knots 0 0 0 1 2 3 3 3
  line L134 (134.3942, -60.3531) -> (134.3942, -60.3825)
  spline S166 degree 2 poles (134.3942, -60.3825) (134.3942, -60.4706) (134.4529, -60.5293) (134.4921, -60.5195) knots 0 0 0 1 2 2 2
  spline S167 degree 2 poles (134.4921, -60.5195) (134.5214, -60.5293) (134.5802, -60.4608) (134.5802, -60.3825) knots 0 0 0 1 2 2 2
  line L135 (134.5802, -60.3825) -> (134.5802, -58.2686)
  spline S168 degree 2 poles (134.5802, -58.2686) (134.5802, -58.1805) (134.5214, -58.1414) (134.4921, -58.1414) knots 0 0 0 1 2 2 2
  spline S169 degree 2 poles (134.4921, -58.1414) (134.4529, -58.1414) (134.3942, -58.1805) (134.3942, -58.2686) knots 0 0 0 1 2 2 2
  line L136 (134.3942, -58.2686) -> (134.3942, -58.3762)
  spline S170 degree 2 poles (134.3942, -58.3762) (134.404, -58.7286) (133.7874, -59.1983) (132.2118, -59.4234) (130.7928, -59.4234) knots 0 0 0 1 2 3 3 3
  line L137 (130.7928, -59.4234) -> (124.2261, -59.4234)
  line L138 (124.2261, -59.4234) -> (124.2261, -59.4136)
  line L139 (124.2261, -59.4136) -> (134.5019, -57.3682)
  spline S171 degree 2 poles (134.5019, -57.3682) (134.5704, -57.3585) (134.6389, -57.2997) (134.6389, -57.2312) knots 0 0 0 1 2 2 2
  line L140 (134.6389, -57.2312) -> (134.6389, -55.9101)
  spline S172 degree 2 poles (134.6389, -55.9101) (134.6389, -55.8415) (134.5704, -55.7633) (134.4823, -55.7535) knots 0 0 0 1 2 2 2
  line L141 (134.4823, -55.7535) -> (124.2261, -54.0996)
  line L142 (124.2261, -54.0996) -> (124.2261, -54.0702)
  line L143 (124.2261, -54.0702) -> (133.7874, -54.0702)
  spline S173 degree 2 poles (133.7874, -54.0702) (134.1593, -54.0702) (134.404, -54.1191) (134.3942, -54.2268) knots 0 0 0 1 2 2 2
  line L144 (134.3942, -54.2268) -> (134.3942, -54.6574)
  spline S174 degree 2 poles (134.3942, -54.6574) (134.3942, -54.7357) (134.4529, -54.7944) (134.4823, -54.7944) knots 0 0 0 1 2 2 2
  spline S175 degree 2 poles (134.4823, -54.7944) (134.5214, -54.7944) (134.5802, -54.7357) (134.5802, -54.6574) knots 0 0 0 1 2 2 2
  line L145 (134.5802, -54.6574) -> (134.5802, -51.1636)
  spline S176 degree 2 poles (134.5802, -51.1636) (134.5802, -51.0853) (134.5214, -51.0266) (134.4921, -51.0266) knots 0 0 0 1 2 2 2
  spline S177 degree 2 poles (126.7901, -43.1583) (125.5472, -43.1778) (124.1673, -44.1174) (123.6389, -45.5168) (123.6487, -46.2214) knots 0 0 0 1 2 3 3 3
  line L146 (123.6487, -46.2214) -> (123.6487, -50.2926)
  spline S178 degree 2 poles (123.6487, -50.2926) (123.6487, -50.3709) (123.7074, -50.4296) (123.7465, -50.4296) knots 0 0 0 1 2 2 2
  spline S179 degree 2 poles (123.7465, -50.4296) (123.7759, -50.4394) (123.8346, -50.3807) (123.8346, -50.2926) knots 0 0 0 1 2 2 2
  line L147 (123.8346, -50.2926) -> (123.8346, -49.862)
  spline S180 degree 2 poles (123.8346, -49.862) (123.8248, -49.7544) (124.0695, -49.7054) (124.4414, -49.7054) knots 0 0 0 1 2 2 2
  line L148 (124.4414, -49.7054) -> (133.7972, -49.7054)
  spline S181 degree 2 poles (133.7972, -49.7054) (134.1691, -49.7054) (134.404, -49.7544) (134.3942, -49.862) knots 0 0 0 1 2 2 2
  line L149 (134.3942, -49.862) -> (134.3942, -50.2926)
  spline S182 degree 2 poles (134.3942, -50.2926) (134.3942, -50.3807) (134.4529, -50.4394) (134.4921, -50.4296) knots 0 0 0 1 2 2 2
  spline S183 degree 2 poles (134.4921, -50.4296) (134.5214, -50.4296) (134.5802, -50.3709) (134.5802, -50.2926) knots 0 0 0 1 2 2 2
  line L150 (134.5802, -50.2926) -> (134.5802, -46.4857)
  spline S184 degree 2 poles (134.5802, -46.4857) (134.5802, -46.4074) (134.5214, -46.3487) (134.4921, -46.3487) knots 0 0 0 1 2 2 2
  spline S185 degree 2 poles (134.4921, -46.3487) (134.4529, -46.3389) (134.3942, -46.3976) (134.3942, -46.4857) knots 0 0 0 1 2 2 2
  line L151 (134.3942, -46.4857) -> (134.3942, -47.2294)
  spline S186 degree 2 poles (134.3942, -47.2294) (134.404, -47.3371) (134.1691, -47.386) (133.7972, -47.386) knots 0 0 0 1 2 2 2
  line L152 (133.7972, -47.386) -> (129.9316, -47.386)
  spline S187 degree 2 poles (129.9316, -47.386) (129.9022, -47.386) (129.8337, -47.3371) (129.8239, -47.2588) knots 0 0 0 1 2 2 2
  line L153 (129.8239, -47.2588) -> (129.8239, -46.0844)
  spline S188 degree 2 poles (129.8239, -46.0844) (129.8337, -45.3211) (129.2074, -43.9901) (127.8666, -43.1681) (126.7901, -43.1583) knots 0 0 0 1 2 3 3 3
  spline S189 degree 2 poles (126.751, -45.5853) (127.8568, -45.5853) (129.1193, -45.7811) (129.638, -46.2704) (129.6282, -46.7206) knots 0 0 0 1 2 3 3 3
  line L154 (129.6282, -46.7206) -> (129.6282, -47.2784)
  spline S190 degree 2 poles (129.6282, -47.2784) (129.6282, -47.3469) (129.5695, -47.386) (129.5401, -47.386) knots 0 0 0 1 2 2 2
  line L155 (129.5401, -47.386) -> (123.9618, -47.386)
  spline S191 degree 2 poles (123.9618, -47.386) (123.9227, -47.386) (123.864, -47.3273) (123.864, -47.2588) knots 0 0 0 1 2 2 2
  line L156 (123.864, -47.2588) -> (123.864, -46.7206)
  spline S192 degree 2 poles (123.864, -46.7206) (123.864, -46.3095) (124.3924, -45.8104) (125.6549, -45.5853) (126.751, -45.5853) knots 0 0 0 1 2 3 3 3
  line L157 (134.4529, -35.701) -> (130.6362, -35.701)
  spline S193 degree 2 poles (130.6362, -35.701) (130.5579, -35.701) (130.4894, -35.7597) (130.4992, -35.8086) knots 0 0 0 1 2 2 2
  spline S194 degree 2 poles (130.4992, -35.8086) (130.4894, -35.8576) (130.5579, -35.9065) (130.6362, -35.9065) knots 0 0 0 1 2 2 2
  line L158 (130.6362, -35.9065) -> (130.8026, -35.9065)
  spline S195 degree 2 poles (130.8026, -35.9065) (131.1353, -35.8967) (132.2901, -36.1805) (133.5036, -36.8362) (134.3453, -37.9519) (134.3648, -38.7739) knots 0 0 0 1 2 3 4 4 4
  line L159 (134.3648, -38.7739) -> (134.3648, -39.3611)
  spline S196 degree 2 poles (134.3648, -39.3611) (134.3648, -39.4296) (134.3257, -39.4688) (134.2866, -39.4688) knots 0 0 0 1 2 2 2
  line L160 (134.2866, -39.4688) -> (129.041, -39.4688)
  spline S197 degree 2 poles (129.041, -39.4688) (129.0019, -39.4688) (128.9431, -39.4101) (128.9431, -39.3415) knots 0 0 0 1 2 2 2
  line L161 (128.9431, -39.3415) -> (128.9431, -39.1165)
  spline S198 degree 2 poles (128.9431, -39.1165) (128.9529, -38.725) (129.501, -38.0693) (130.3524, -37.6681) (130.8221, -37.6681) knots 0 0 0 1 2 3 3 3
  line L162 (130.8221, -37.6681) -> (130.9298, -37.6681)
  spline S199 degree 2 poles (130.9298, -37.6681) (131.0179, -37.6681) (131.0668, -37.6093) (131.0668, -37.5604) knots 0 0 0 1 2 2 2
  spline S200 degree 2 poles (131.0668, -37.5604) (131.0668, -37.5115) (131.0179, -37.4625) (130.9298, -37.4625) knots 0 0 0 1 2 2 2
  line L163 (130.9298, -37.4625) -> (126.7803, -37.4625)
  spline S201 degree 2 poles (126.7803, -37.4625) (126.702, -37.4625) (126.6335, -37.5115) (126.6433, -37.5604) knots 0 0 0 1 2 2 2
  spline S202 degree 2 poles (126.6433, -37.5604) (126.6335, -37.6093) (126.702, -37.6681) (126.7803, -37.6681) knots 0 0 0 1 2 2 2
  line L164 (126.7803, -37.6681) -> (126.8978, -37.6681)
  spline S203 degree 2 poles (126.8978, -37.6681) (127.3577, -37.6681) (128.2092, -38.0693) (128.7474, -38.725) (128.7572, -39.1165) knots 0 0 0 1 2 3 3 3
  line L165 (128.7572, -39.1165) -> (128.7572, -39.3611)
  spline S204 degree 2 poles (128.7572, -39.3611) (128.7572, -39.4296) (128.7083, -39.4688) (128.6691, -39.4688) knots 0 0 0 1 2 2 2
  line L166 (128.6691, -39.4688) -> (123.9618, -39.4688)
  spline S205 degree 2 poles (123.9618, -39.4688) (123.9129, -39.4688) (123.864, -39.4101) (123.864, -39.3415) knots 0 0 0 1 2 2 2
  line L167 (123.864, -39.3415) -> (123.864, -38.6761)
  spline S206 degree 2 poles (123.864, -38.6761) (123.8835, -37.9714) (124.872, -36.9243) (126.428, -36.3371) (127.2892, -36.3371) knots 0 0 0 1 2 3 3 3
  line L168 (127.2892, -36.3371) -> (127.4947, -36.3371)
  spline S207 degree 2 poles (127.4947, -36.3371) (127.5828, -36.3371) (127.6318, -36.2784) (127.6318, -36.2294) knots 0 0 0 1 2 2 2
  spline S208 degree 2 poles (127.6318, -36.2294) (127.6318, -36.1903) (127.573, -36.1218) (127.4947, -36.1218) knots 0 0 0 1 2 2 2
  line L169 (127.4947, -36.1218) -> (123.7563, -36.1218)
  spline S209 degree 2 poles (123.7563, -36.1218) (123.6976, -36.1218) (123.6487, -36.1903) (123.6487, -36.249) knots 0 0 0 1 2 2 2
  line L170 (123.6487, -36.249) -> (123.6487, -42.3754)
  spline S210 degree 2 poles (123.6487, -42.3754) (123.6487, -42.4536) (123.7074, -42.5124) (123.7465, -42.5124) knots 0 0 0 1 2 2 2
  spline S211 degree 2 poles (123.7465, -42.5124) (123.7759, -42.5222) (123.8346, -42.4634) (123.8346, -42.3754) knots 0 0 0 1 2 2 2
  line L171 (123.8346, -42.3754) -> (123.8346, -41.9448)
  spline S212 degree 2 poles (123.8346, -41.9448) (123.8248, -41.8371) (124.0695, -41.7882) (124.4414, -41.7882) knots 0 0 0 1 2 2 2
  line L172 (124.4414, -41.7882) -> (133.7972, -41.7882)
  spline S213 degree 2 poles (133.7972, -41.7882) (134.1691, -41.7882) (134.404, -41.8371) (134.3942, -41.9448) knots 0 0 0 1 2 2 2
  line L173 (134.3942, -41.9448) -> (134.3942, -42.3754)
  spline S214 degree 2 poles (134.3942, -42.3754) (134.3942, -42.4634) (134.4529, -42.5222) (134.4921, -42.5124) knots 0 0 0 1 2 2 2
  spline S215 degree 2 poles (134.4921, -42.5124) (134.5214, -42.5124) (134.5802, -42.4536) (134.5802, -42.3754) knots 0 0 0 1 2 2 2
  line L174 (134.5802, -42.3754) -> (134.5802, -35.8086)
  spline S216 degree 2 poles (134.5802, -35.8086) (134.5802, -35.7499) (134.5214, -35.701) (134.4529, -35.701) knots 0 0 0 1 2 2 2
  spline S217 degree 2 poles (133.856, -26.8834) (133.8266, -26.9421) (133.9049, -27.0106) (133.9636, -27.0399) knots 0 0 0 1 2 2 2
  spline S218 degree 2 poles (133.9636, -27.0399) (134.1398, -27.0987) (134.4138, -27.3531) (134.4236, -27.5293) knots 0 0 0 1 2 2 2
  spline S219 degree 2 poles (134.4236, -27.5293) (134.4138, -27.7739) (133.9734, -27.9012) (133.6015, -27.8914) knots 0 0 0 1 2 2 2
  spline S220 degree 2 poles (133.6015, -27.8914) (133.2296, -27.8914) (132.2216, -27.8718) (131.7519, -27.8718) knots 0 0 0 1 2 2 2
  spline S221 degree 2 poles (131.7519, -27.8718) (130.7145, -27.8914) (129.4814, -28.6547) (128.9138, -29.8095) (128.8746, -30.4163) knots 0 0 0 1 2 3 3 3
  line L175 (128.8746, -30.4163) -> (128.8551, -30.4163)
  spline S222 degree 2 poles (128.8551, -30.4163) (128.7866, -29.7508) (128.1211, -28.6449) (127.0348, -27.9794) (126.3106, -27.9697) knots 0 0 0 1 2 3 3 3
  spline S223 degree 2 poles (126.3106, -27.9697) (125.3417, -27.9892) (124.1673, -28.8015) (123.6487, -30.064) (123.6487, -30.749) knots 0 0 0 1 2 3 3 3
  line L176 (123.6487, -30.749) -> (123.6487, -34.7615)
  spline S224 degree 2 poles (123.6487, -34.7615) (123.6487, -34.8398) (123.7074, -34.8985) (123.7465, -34.8985) knots 0 0 0 1 2 2 2
  spline S225 degree 2 poles (123.7465, -34.8985) (123.7759, -34.8985) (123.8248, -34.8496) (123.8248, -34.7615) knots 0 0 0 1 2 2 2
  line L177 (123.8248, -34.7615) -> (123.8248, -34.3113)
  spline S226 degree 2 poles (123.8248, -34.3113) (123.815, -34.2036) (124.0793, -34.1547) (124.4414, -34.1547) knots 0 0 0 1 2 2 2
  line L178 (124.4414, -34.1547) -> (133.7874, -34.1547)
  spline S227 degree 2 poles (133.7874, -34.1547) (134.1495, -34.1547) (134.404, -34.2036) (134.3942, -34.3113) knots 0 0 0 1 2 2 2
  line L179 (134.3942, -34.3113) -> (134.3942, -34.7615)
  spline S228 degree 2 poles (134.3942, -34.7615) (134.3942, -34.8496) (134.4529, -34.8985) (134.4823, -34.8985) knots 0 0 0 1 2 2 2
  spline S229 degree 2 poles (134.4823, -34.8985) (134.5214, -34.8985) (134.5802, -34.8398) (134.5802, -34.7615) knots 0 0 0 1 2 2 2
  line L180 (134.5802, -34.7615) -> (134.5802, -31.3362)
  spline S230 degree 2 poles (134.5802, -31.3362) (134.5802, -31.2579) (134.5214, -31.1992) (134.4823, -31.1992) knots 0 0 0 1 2 2 2
  spline S231 degree 2 poles (134.4823, -31.1992) (134.4529, -31.1992) (134.3942, -31.2481) (134.3942, -31.3362) knots 0 0 0 1 2 2 2
  line L181 (134.3942, -31.3362) -> (134.3942, -31.7864)
  spline S232 degree 2 poles (134.3942, -31.7864) (134.404, -31.894) (134.1495, -31.943) (133.7874, -31.943) knots 0 0 0 1 2 2 2
  line L182 (133.7874, -31.943) -> (129.041, -31.943)
  spline S233 degree 2 poles (129.041, -31.943) (128.9921, -31.943) (128.9334, -31.8843) (128.9334, -31.8157) knots 0 0 0 1 2 2 2
  line L183 (128.9334, -31.8157) -> (128.9334, -31.1209)
  spline S234 degree 2 poles (128.9334, -31.1209) (128.9138, -30.6316) (129.5793, -30.0835) (130.5285, -30.0738) knots 0 0 0 1 2 2 2
  spline S235 degree 2 poles (130.5285, -30.0738) (131.0962, -30.064) (132.1433, -30.0835) (132.7207, -30.0933) knots 0 0 0 1 2 2 2
  spline S236 degree 2 poles (132.7207, -30.0933) (133.6504, -30.0835) (134.7563, -29.056) (134.7661, -28.0969) knots 0 0 0 1 2 2 2
  spline S237 degree 2 poles (134.7661, -28.0969) (134.7563, -27.5782) (134.3648, -26.9617) (134.0419, -26.8442) knots 0 0 0 1 2 2 2
  spline S238 degree 2 poles (134.0419, -26.8442) (133.9636, -26.8149) (133.8755, -26.8246) (133.856, -26.8834) knots 0 0 0 1 2 2 2
  spline S239 degree 2 poles (126.3302, -30.0738) (127.6905, -30.064) (128.767, -30.5337) (128.7474, -31.1209) knots 0 0 0 1 2 2 2
  line L184 (128.7474, -31.1209) -> (128.7474, -31.8353)
  spline S240 degree 2 poles (128.7474, -31.8353) (128.7474, -31.9038) (128.6985, -31.943) (128.6593, -31.943) knots 0 0 0 1 2 2 2
  line L185 (128.6593, -31.943) -> (123.9618, -31.943)
  spline S241 degree 2 poles (123.9618, -31.943) (123.9129, -31.943) (123.8542, -31.8843) (123.8542, -31.8157) knots 0 0 0 1 2 2 2
  line L186 (123.8542, -31.8157) -> (123.8542, -31.1405)
  spline S242 degree 2 poles (123.8542, -31.1405) (123.8346, -30.5827) (124.9992, -30.0738) (126.3302, -30.0738) knots 0 0 0 1 2 2 2
  spline S243 degree 2 poles (134.4921, -22.7045) (134.4529, -22.6948) (134.3942, -22.7535) (134.3942, -22.8415) knots 0 0 0 1 2 2 2
  line L187 (134.3942, -22.8415) -> (134.3942, -23.2722)
  spline S244 degree 2 poles (134.3942, -23.2722) (134.404, -23.3798) (134.1691, -23.4287) (133.7972, -23.4287) knots 0 0 0 1 2 2 2
  line L188 (133.7972, -23.4287) -> (124.4414, -23.4287)
  spline S245 degree 2 poles (124.4414, -23.4287) (124.0695, -23.4287) (123.8248, -23.3798) (123.8346, -23.2722) knots 0 0 0 1 2 2 2
  line L189 (123.8346, -23.2722) -> (123.8346, -22.8415)
  spline S246 degree 2 poles (123.8346, -22.8415) (123.8346, -22.7535) (123.7759, -22.6948) (123.7465, -22.7045) knots 0 0 0 1 2 2 2
  spline S247 degree 2 poles (123.7465, -22.7045) (123.7074, -22.7045) (123.6487, -22.7633) (123.6487, -22.8415) knots 0 0 0 1 2 2 2
  line L190 (123.6487, -22.8415) -> (123.6487, -26.3353)
  spline S248 degree 2 poles (123.6487, -26.3353) (123.6487, -26.4136) (123.7074, -26.4723) (123.7465, -26.4723) knots 0 0 0 1 2 2 2
  spline S249 degree 2 poles (123.7465, -26.4723) (123.7759, -26.4821) (123.8346, -26.4234) (123.8346, -26.3353) knots 0 0 0 1 2 2 2
  line L191 (123.8346, -26.3353) -> (123.8346, -25.9047)
  spline S250 degree 2 poles (123.8346, -25.9047) (123.8248, -25.7971) (124.0695, -25.7481) (124.4414, -25.7481) knots 0 0 0 1 2 2 2
  line L192 (124.4414, -25.7481) -> (133.7972, -25.7481)
  spline S251 degree 2 poles (133.7972, -25.7481) (134.1691, -25.7481) (134.404, -25.7971) (134.3942, -25.9047) knots 0 0 0 1 2 2 2
  line L193 (134.3942, -25.9047) -> (134.3942, -26.3353)
  spline S252 degree 2 poles (134.3942, -26.3353) (134.3942, -26.4234) (134.4529, -26.4821) (134.4921, -26.4723) knots 0 0 0 1 2 2 2
  spline S253 degree 2 poles (134.4921, -26.4723) (134.5214, -26.4723) (134.5802, -26.4136) (134.5802, -26.3353) knots 0 0 0 1 2 2 2
  line L194 (134.5802, -26.3353) -> (134.5802, -22.8415)